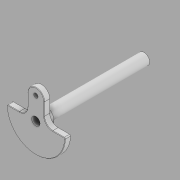
# Autodesk Inventor part: Crankshaft
Saved by Autodesk Inventor 2020 (Build 240168000, 168)
## iProperties
Created: 2019-10-15
Part Number: Crankshaft
Material: Genérico
Document SubType Name: Modeling
Designer: gerar
Density: 1 g/cm^3
Appearance: Valor por defecto
Author: gerar
Autodesk Inventor part; units mm, degrees
ref_plane "YZ Plane" through (0, 0, 0) normal (1, 0, 0) x (0, 1, 0)
ref_plane "XZ Plane" through (0, 0, 0) normal (0, 1, 0) x (-1, 0, 0)
ref_plane "XY Plane" through (0, 0, 0) normal (0, 0, 1) x (1, 0, 0)
sketch "Boceto1" plane through (0, 0, 0) normal (0, 0, 1) x (1, 0, 0)
  arc A0 (-16.6573, -0.6174) -> (16.6573, -0.6174) centre (0, 0) ccw
  circle A1 centre (0, 0) radius 2.3813
  circle A2 centre (0, 0) radius 4.7625 construction
  line L0 (-23.5039, 0) -> (23.5039, 0) construction
  arc A3 (4.7625, 11.9062) -> (-4.7625, 11.9062) centre (0, 11.9062) ccw
  arc A4 (-9.525, 0) -> (-4.7625, 4.7625) centre (-9.525, 4.7625) ccw
  arc A5 (4.7625, 4.7625) -> (9.525, 0) centre (9.525, 4.7625) ccw
  line L1 (-16.0624, 0) -> (-9.525, 0)
  line L2 (16.0624, 0) -> (9.525, 0)
  line L3 (-4.7625, 11.9062) -> (-4.7625, 4.7625)
  line L4 (4.7625, 11.9062) -> (4.7625, 4.7625)
  arc A6 (-16.0624, 0) -> (-16.6573, -0.6174) centre (-16.0624, -0.5953) ccw
  arc A7 (16.6573, -0.6174) -> (16.0624, 0) centre (16.0624, -0.5953) ccw
  dimension "d0" = 33.3375
  dimension "d2" = 4.7625
  dimension "d3" = 9.525
  dimension "d6" = 9.525
  dimension "d21" = 4.7625
  dimension "d22" = 1.1906
  dimension "d23" = 1.1906
  constraints: 12 point on circle, 11 tangent, 8 centre point, 8 end point, 3 coincident, 2 equal radius, 2 vertical, 1 point on line
  measures "d0" diameter of A0
  measures "d2" diameter of A1
  measures "d3" diameter of A2
  measures "d6" diameter of A3
  measures "d21" radius of A4
  measures "d22" diameter of A6
  measures "d23" diameter of A7
extrude "Extrusión1" add sketch "Boceto1" against normal blind 3.175
sketch "Boceto2" plane through (0, 0, 0) normal (0, 0, 1) x (1, 0, 0)
  line L0 (0, 0) -> (0, 12.7) construction
  dimension "d9" = 12.7
  constraints: 2 end point, 1 coincident, 1 vertical
  measures "d9" distance of L0.start L0.end
hole "Agujero1" at (0, 12.7, 0) direction (0, 0, -1) diameter 2.4867 end through all thread size "5-40 UNC" class "2B" standard "ANSI Unified Screw Threads"
sketch "Boceto3" plane through (0, 0, -3.175) normal (0, 0, -1) x (-1, 0, 0)
  circle A0 centre (0, 0) radius 4.7625
  circle A1 centre (0, 0) radius 2.3813
  dimension "d17" = 9.525
  dimension "d18" = 4.7625
  constraints: 2 centre point, 2 coincident
  measures "d17" diameter of A0
  measures "d18" diameter of A1
extrude "Extrusión2" add sketch "Boceto3" along normal blind 2.3813
sketch "Boceto4" plane through (0, 0, -5.5563) normal (0, 0, -1) x (-1, 0, 0)
  circle A0 centre (0, 0) radius 3.175
  dimension "d24" = 6.35
  constraints: 1 centre point, 1 coincident
  measures "d24" diameter of A0
extrude "Extrusión3" add sketch "Boceto4" along normal blind 56.3563
fillet "Empalme1" radius 0.254 10 edges at (-4.7625, 8.3344, 0) (-6.1574, 1.3949, 0) (-12.7937, 0, 0) (-16.4911, -0.1822, 0) (0, -16.6688, 0) (16.4911, -0.1822, 0) (12.7937, 0, 0) (6.1574, 1.3949, 0) (4.7625, 8.3344, 0) (0, 16.6687, 0)
equation "\"d22\" = 0.25 * d21"
equation "\"d23\" = 0.25 * d21"
